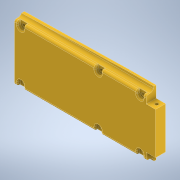
# Autodesk Inventor part: BodyStructure Side
Saved by Autodesk Inventor 2022.2 (Build 262287030, 287C)
## iProperties
Created: 2022-01-14
Part Number: BodyStructure Side
Material: Generic
Document SubType Name: Modeling
Designer: Jochen
Density: 1 g/cm^3
Appearance: Default
Author: Jochen
Autodesk Inventor part; units mm, degrees
ref_plane "YZ Plane" through (0, 0, 0) normal (1, 0, 0) x (0, 1, 0)
ref_plane "XZ Plane" through (0, 0, 0) normal (0, 1, 0) x (-1, 0, 0)
ref_plane "Work Plane1" through (0, 0, 50) normal (0, 0, 1) x (1, 0, 0)
sketch "Sketch1" plane through (0, 0, 50) normal (0, 0, 1) x (1, 0, 0)
  line L0 (0, -20) -> (0, 20)
  line L1 (0, 20) -> (-9, 20)
  line L2 (-9, -31) -> (-32, -31)
  line L3 (-33.565, -30.9847) -> (-135, -29)
  line L4 (-135, -29) -> (-135, 29)
  line L5 (-135, 29) -> (-33.565, 30.9847)
  line L6 (-32, 31) -> (-9, 31)
  line L7 (-9, 31) -> (-9, 20)
  line L8 (-9, -20) -> (0, -20)
  line L9 (0, -68.6) -> (0, 68.6) construction
  line L10 (-166.1569, 0) -> (27.6928, 0) construction
  line L11 (-9, -20) -> (-9, -31)
  arc A0 (-33.565, -30.9847) -> (-32, -31) centre (-32, 49) ccw
  arc A1 (-32, 31) -> (-33.565, 30.9847) centre (-32, -49) ccw
  line L12 (-32, -31) -> (-138.4641, -31) construction
  point P0 (0, 0)
  point P1 (-9, 20)
  point P2 (-32.7825, -30.9962)
  point P3 (-9, -25.5)
  dimension "d2" = 135
  dimension "d3" = 40
  dimension "d4" = 9
  dimension "d6" = 80
  dimension "d7" = 58
  dimension "d8" = 62
  dimension "d9" = 23
  dimension "d71" = 32
  dimension "d72" = 4
  dimension "d73" = 126
  constraints: 22 end point, 5 point on circle, 4 perpendicular, 4 tangent, 3 point on line, 2 centre point, 2 parallel, 1 equal radius, 1 horizontal, 1 midpoint, 1 vertical, 4 other
  measures "d2" distance between parallel lines of L4 L9
  measures "d3" distance of L0.start L0.end
  measures "d4" distance between parallel lines of L9 L11
  measures "d6" radius of A0
  measures "d7" distance of L3.end L4.end
  measures "d8" distance between parallel lines of L6 L2
  measures "d9" distance of L2.start L2.end
  measures "d71" distance from line of L2.end L9
  measures "d72" distance of L12.end L3.end
  measures "d73" distance from line of L4 point (-9, -25.5)
extrude "Extrusion1" add sketch "Sketch1" along normal blind 10
sketch "Sketch2" plane through (0, 0, 50) normal (0, 0, 1) x (1, 0, 0)
  circle A0 centre (-55, -23.5) radius 1.5
  circle A1 centre (-15, -23.5) radius 1.5
  circle A2 centre (-55, 23.5) radius 1.5
  circle A3 centre (-15, 23.5) radius 1.5
  line L0 (-4, -10) -> (-4, 10) construction
  line L1 (-5.5, -10) -> (-5.5, 10)
  line L2 (-2.5, 10) -> (-2.5, -10)
  arc A4 (-5.5, -10) -> (-2.5, -10) centre (-4, -10) ccw
  arc A5 (-2.5, 10) -> (-5.5, 10) centre (-4, 10) ccw
  line L3 (-135, -11) -> (-127, -11)
  line L4 (-125, -9) -> (-125, 9)
  line L5 (-127, 11) -> (-135, 11)
  line L6 (-135, 11) -> (-135, -11)
  arc A6 (-127, -11) -> (-125, -9) centre (-127, -9) ccw
  arc A7 (-125, 9) -> (-127, 11) centre (-127, 9) ccw
  line L7 (0, -20) -> (-9, -20) projected
  line L8 (-9, -20) -> (-9, -31) projected
  line L9 (-9, -31) -> (-32, -31) projected
  arc A8 (-33.565, -30.9847) -> (-32, -31) centre (-32, 49) ccw projected
  line L10 (-33.565, -30.9847) -> (-135, -29) projected
  line L11 (-135, -29) -> (-135, 29) projected
  line L12 (-135, 29) -> (-33.565, 30.9847) projected
  arc A9 (-32, 31) -> (-33.565, 30.9847) centre (-32, -49) ccw projected
  line L13 (-32, 31) -> (-9, 31) projected
  line L14 (-9, 31) -> (-9, 20) projected
  line L15 (-9, 20) -> (0, 20) projected
  line L16 (0, 20) -> (0, -20) projected
  line L17 (0, -20) -> (-9, -20) projected
  line L18 (-9, -20) -> (-9, -31) projected
  line L19 (-9, -31) -> (-32, -31) projected
  line L20 (-32, 31) -> (-9, 31) projected
  line L21 (-9, 31) -> (-9, 20) projected
  line L22 (-9, 20) -> (0, 20) projected
  line L23 (0, 20) -> (0, -20) projected
  line L24 (0, -68.6) -> (0, 68.6) construction
  line L25 (-162, 0) -> (27, 0) construction
  line L26 (-135, 29) -> (-135, -29) construction
  arc A10 (-52, -23.5) -> (-58, -23.5) centre (-55, -23.5) ccw
  arc A11 (-12, -23.5) -> (-18, -23.5) centre (-15, -23.5) ccw
  arc A12 (-58, 23.5) -> (-52, 23.5) centre (-55, 23.5) ccw
  arc A13 (-18, 23.5) -> (-12, 23.5) centre (-15, 23.5) ccw
  line L27 (-7, -19) -> (-7, 19)
  arc A14 (-19.5, 23.5) -> (-15, 19) centre (-15, 23.5) ccw
  line L28 (-19.5, 23.5) -> (-50.5, 23.5)
  line L29 (-54, 19.1125) -> (-54, -19.1125)
  line L30 (-50.5, -23.5) -> (-19.5, -23.5)
  arc A15 (-15, -19) -> (-19.5, -23.5) centre (-15, -23.5) ccw
  line L31 (-15, -19) -> (-7, -19)
  line L32 (-55, -23.5) -> (-55, 23.5) construction
  line L33 (-56, -19.1125) -> (-56, 19.1125)
  arc A16 (-50.5, -23.5) -> (-54, -19.1125) centre (-55, -23.5) ccw
  arc A17 (-89.9137, 21.9371) -> (-89.9137, 21.9371) centre (-89.5655, 22.3741) ccw
  line L34 (-123, 22.3024) -> (-123, -22.2576)
  line L35 (-58, -23.5) -> (-58, -30.5066)
  line L36 (-52, -23.5) -> (-52, -30.624)
  line L37 (-135, -29) -> (-33.565, -30.9847) projected
  line L38 (-18, -23.5) -> (-18, -31)
  line L39 (-12, -23.5) -> (-12, -31)
  line L40 (-12, 23.5) -> (-12, 31)
  line L41 (-9, 31) -> (-32, 31) projected
  line L42 (-18, 23.5) -> (-18, 31)
  line L43 (-52, 23.5) -> (-52, 30.624)
  line L44 (-58, 23.5) -> (-58, 30.5066)
  line L45 (-33.565, 30.9847) -> (-135, 29) projected
  arc A18 (-33.565, -30.9847) -> (-32, -31) centre (-32, 49) ccw projected
  line L46 (-33.565, -30.9847) -> (-135, -29) projected
  line L47 (-135, -29) -> (-135, 29) projected
  line L48 (-135, 29) -> (-33.565, 30.9847) projected
  arc A19 (-32, 31) -> (-33.565, 30.9847) centre (-32, -49) ccw projected
  arc A20 (-49.3875, 23.2839) -> (-49.3875, 23.2839) centre (-49.8289, 22.9413) ccw
  arc A21 (-56, -19.1125) -> (-59.4991, -23.412) centre (-55, -23.5) ccw
  arc A22 (-59.5, 23.5) -> (-56, 19.1125) centre (-55, 23.5) ccw
  arc A23 (-54, 19.1125) -> (-50.5, 23.5) centre (-55, 23.5) ccw
  arc A24 (-9, 19) -> (-9, 19) centre (-9, 20) ccw
  line L49 (-19.5, 23.5) -> (-19.5, 23.5)
  line L50 (-50.5, 23.5) -> (-50.5, 23.5)
  line L51 (-59.5, 23.5) -> (-59.5, 23.5)
  line L52 (-7, 19) -> (-15, 19)
  line L53 (0, 20) -> (-9, 20) projected
  line L54 (-123, -22.2576) -> (-59.5009, -23.5)
  line L55 (-59.5, 23.5) -> (-123, 22.3024)
  line L56 (-59.4991, -23.412) -> (-59.5009, -23.5)
  line L57 (-50.5, -23.5) -> (-50.5, -23.5)
  circle A25 centre (-129, -23.5) radius 1.5
  arc A26 (-126, -23.5) -> (-132, -23.5) centre (-129, -23.5) ccw
  line L58 (-126, -23.5) -> (-126, -29.1761)
  line L59 (-132, -23.5) -> (-132, -29.0587)
  circle A27 centre (-129, 23.5) radius 1.5
  arc A28 (-132, 23.5) -> (-126, 23.5) centre (-129, 23.5) ccw
  line L60 (-126, 23.5) -> (-126, 29.1761)
  line L61 (-132, 23.5) -> (-132, 29.0587)
  line L62 (-15, 23.5) -> (-129, 23.5) construction
  point P0 (0, 0)
  point P1 (-4, 0)
  point P2 (-135, 0)
  point P3 (-54.5017, 19)
  point P4 (-52, -30.624)
  point P5 (-58, 30.5066)
  point P6 (-50.7819, 25.4474)
  point P7 (-132, 29.0587)
  dimension "d12" = 2
  dimension "d13" = 22
  dimension "d14" = 10
  dimension "d15" = 3
  dimension "d16" = 6
  dimension "d17" = 47
  dimension "d18" = 47
  dimension "d20" = 55
  dimension "d21" = 15
  dimension "d22" = 4
  dimension "d23" = 20
  dimension "d24" = 1.5
  dimension "d25" = 3
  dimension "d27" = 1.5
  dimension "d29" = 2
  dimension "d30" = 2
  dimension "d77" = 1.5
  dimension "d91" = 6
  constraints: 76 end point, 38 point on circle, 25 centre point, 23 tangent, 22 point on line, 15 equal radius, 13 vertical, 10 coincident, 9 parallel, 4 perpendicular, 3 equal length, 3 horizontal, 3 midpoint, 2 collinear, 2 symmetric about line, 1 concentric, 5 other
  measures "d12" radius of A6
  measures "d13" distance of L5.end L3.start
  measures "d14" distance between parallel lines of L11 L4
  measures "d15" diameter of A1
  measures "d16" diameter of A11
  measures "d17" distance of A2.centre A0.centre
  measures "d18" distance of A3.centre A1.centre
  measures "d20" distance from line of L16 A0.centre
  measures "d21" distance from line of L24 A1.centre
  measures "d22" distance between parallel lines of L24 L0
  measures "d23" distance of L0.start L0.end
  measures "d24" radius of A4
  measures "d25" distance between parallel lines of L0 L27
  measures "d27" radial gap between concentric circles of A13 A14
  measures "d29" distance between parallel lines of L29 L33
  measures "d30" distance between parallel lines of L34 L4
  measures "d77" radial gap between concentric circles of A23 A12
  measures "d91" distance from line of L47 A25.centre
extrude "Extrusion2" cut sketch "Sketch2" along normal blind 9 contours L1 A5 L2 A4 | L6 L5 A7 L4 A6 L3 | A20 | L52 L27 L31 A15 L30 A16 L29 A23 L28 A14 | A17 | A21 L56 L54 L34 L55 A22 L33 | A25 | A27
sketch "Sketch3" plane through (0, 0, 0) normal (1, 0, 0) x (0, 1, 0)
  line L0 (0, -12.0828) -> (0, 72.4971) construction
  line L1 (-43.4, 0) -> (43.4, 0) construction
  line L2 (-31, 50.5602) -> (-20, 50.5602) construction
  line L3 (-20, 50) -> (-20, 60) construction
  line L4 (-31.0008, 50) -> (-30.9977, 60) construction
  line L5 (20, 50) -> (31, 50) construction
  line L6 (-31, 50) -> (-31, 52.5)
  line L7 (-27, 53.9559) -> (-27, 58)
  line L8 (-31, 52.5) -> (-27, 53.9559)
  line L9 (-25, 60) -> (25, 60)
  line L10 (27, 58) -> (27, 53.9559)
  line L11 (30.9847, 50) -> (20, 50) projected
  line L12 (27, 53.9559) -> (31, 52.5)
  line L13 (31, 50) -> (-31, 50)
  line L14 (31, 52.5) -> (31, 50)
  line L15 (20, 60) -> (20, 50) construction
  line L16 (20, 50) -> (-20, 50) construction
  line L17 (-20, 50) -> (-20, 60) construction
  line L18 (-20, 60) -> (20, 60) construction
  line L19 (20, 60) -> (20, 50) construction
  line L20 (20, 50) -> (-20, 50) construction
  line L21 (-20, 50) -> (-20, 60) construction
  line L22 (-20, 60) -> (20, 60) construction
  line L23 (20, 50) -> (31, 50) construction
  line L24 (31, 50) -> (31, 60) construction
  line L25 (20, 60) -> (31, 60) construction
  line L26 (-20, 50) -> (20, 50) construction
  line L27 (20, 50) -> (20, 60) construction
  line L28 (-20, 60) -> (20, 60) construction
  line L29 (-20, 50) -> (-20, 60) construction
  line L30 (-31, 50) -> (-20, 50) construction
  line L31 (-31, 60) -> (-20, 60) construction
  line L32 (-31, 50) -> (-31, 60) construction
  arc A0 (-25, 60) -> (-27, 58) centre (-25, 58) ccw
  arc A1 (27, 58) -> (25, 60) centre (25, 58) ccw
  line L33 (-31, 50.5) -> (31, 50.5)
  line L34 (-20, 50) -> (-20, 60) projected
  line L35 (20, 50) -> (20, 60) projected
  point P0 (0, 0)
  point P1 (27, 55.9779)
  dimension "d35" = 20
  dimension "d36" = 54
  dimension "d37" = 2.5
  dimension "d38" = 50
  dimension "d65" = 0.5
  constraints: 20 end point, 6 point on line, 4 point on circle, 4 tangent, 2 centre point, 1 coincident, 1 horizontal, 1 midpoint, 1 parallel, 1 perpendicular, 1 vertical, 5 other
  measures "d35" angle of L2 L8
  measures "d36" distance from line of point (27, 55.978) L7
  measures "d37" distance of L2.start L6.end
  measures "d38" distance of L9.end L9.start
  measures "d65" distance between parallel lines of L13 L33
extrude "Extrusion4" cut sketch "Sketch3" against normal through all contours L6 L8 L7 A0 L9 L34 L33 | L34 L9 L35 L33 | L35 L9 A1 L10 L12 L14 L33 keep common part
extrude "Extrusion5" cut sketch "Sketch2" against normal blind 3 from surface at 10 contours A0 | A1 | A2 | A3 | L59 A26 L58 L10 | L12 L60 A28 L61 | L35 A10 L36 L10 | L12 L43 A12 L44 | L38 A11 L39 L9 | L13 L40 A13 L42 | A25 | A27
extrude "Extrusion6" cut sketch "Sketch2" along normal through all contours A0 | A1 | A2 | A3
fillet "Fillet1" radius 1 42 edges at (-18, 26.4142, 59.4142) (-18, 27, 57.5) (-15, 20.5, 60) (-12, 24.25, 60) (-12, 26.4142, 59.4142) (-12, 27, 57.5) (-18, 24.25, 60) (-58, 27, 57.5) (-58, 24.25, 60) (-55, 20.5, 60) (-52, 24.25, 60) (-52, 26.4142, 59.4142) (-52, 27, 57.5) (-58, 26.4142, 59.4142) (-52, -24.25, 60) (-52, -26.4142, 59.4142) (-52, -27, 57.5) (-58, -24.25, 60) (-58, -26.4142, 59.4142) (-58, -27, 57.5) (-55, -20.5, 60) (-12, -24.25, 60) (-12, -26.4142, 59.4142) (-12, -27, 57.5) (-18, -24.25, 60) (-18, -26.4142, 59.4142) (-18, -27, 57.5) (-15, -20.5, 60) (-126, -26.4142, 59.4142) (-126, -27, 57.5) (-129, -20.5, 60) (-132, -24.25, 60) (-132, -26.4142, 59.4142) (-132, -27, 57.5) (-126, -24.25, 60) (-132, 24.25, 60) (-132, 26.4142, 59.4142) (-132, 27, 57.5) (-126, 24.25, 60) (-126, 26.4142, 59.4142) (-126, 27, 57.5) (-129, 20.5, 60)
sketch "Sketch4" plane through (0, 0, 0) normal (0, 1, 0) x (-1, 0, 0)
  line L0 (0, -12) -> (0, 72) construction
  line L1 (10.8, 0) -> (-1.8, 0) construction
  circle A0 centre (4, 55) radius 1.5
  line L2 (5.5, 50.5) -> (5.5, 59) construction
  line L3 (9, 50) -> (0, 50) construction
  line L4 (9, 60) -> (0, 60) construction
  point P0 (0, 0)
  point P1 (5.5, 50)
  point P2 (7, 60)
  dimension "d52" = 3
  dimension "d66" = 5
  constraints: 1 centre point, 1 tangent
  measures "d52" diameter of A0
  measures "d66" distance from line of A0.centre L4
extrude "Extrusion7" cut sketch "Sketch4" along normal through all both and the other way through all
sketch "Sketch5" plane through (0, 0, 0) normal (1, 0, 0) x (0, 1, 0)
  circle A0 centre (15, 55) radius 1.5
  circle A1 centre (-15, 55) radius 1.5
  line L0 (-10, 50) -> (10, 50) projected
  line L1 (0, -12) -> (0, 72) construction
  line L2 (-28, 0) -> (28, 0) construction
  line L3 (-20, 60) -> (20, 60) construction
  point P0 (0, 0)
  dimension "d56" = 3
  dimension "d58" = 30
  dimension "d67" = 5
  constraints: 2 centre point, 1 equal radius, 1 symmetric about line
  measures "d56" diameter of A1
  measures "d58" distance of A0.centre A1.centre
  measures "d67" distance from line of L3 A0.centre
extrude "Extrusion8" cut sketch "Sketch5" along normal blind 10 from surface at -135
fillet "Fillet2" radius 3.5 4 edges at (-72, 27, 53.9559) (-72, -27, 53.9559) (-7, 19, 54.75) (-7, -19, 54.75)
fillet "Fillet2" radius 1 21 edges at (-35, 23.5, 59) (-51.4822, 20.6938, 59) (-54, 0, 59) (-123, 0.0224, 59) (-91.25, 22.9012, 59) (-58.5178, 20.6938, 59) (-18.182, 20.318, 59) (-7, 0, 59) (-11, -19, 59) (-18.182, -20.318, 59) (-35, -23.5, 59) (-51.4822, -20.6938, 59) (-58.4902, -20.6595, 59) (-56, 0, 59) (-54, 19.1125, 54.75) (-56, 19.1125, 54.75) (-56, -19.1125, 54.75) (-54, -19.1125, 54.75) (-50.5, 23.5, 54.75) (-19.5, -23.5, 54.75) (-59.5, 23.5, 54.75)
equation "\"d18\" = d17"
body "Solid1"
